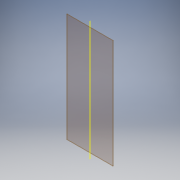
# Autodesk Inventor part: backOfRobot
Saved by Autodesk Inventor 2018.2 (Build 222227000, 227)
## iProperties
Created: 2018-02-09
Part Number: backOfRobot
Material: Polycarbonate, Smoke
Document SubType Name: Modeling
Designer: steele
Density: 1.2 g/cm^3
Appearance: Polycarbonate - Smoked
Author: steele
Autodesk Inventor part; units mm, degrees
ref_plane "XZ Plane" through (0, 0, 0) normal (0, 1, 0) x (-1, 0, 0)
ref_plane "XY Plane" through (0, 0, 0) normal (0, 0, 1) x (1, 0, 0)
sketch "Sketch1" plane through (0, 0, 0) normal (0, 0, 1) x (1, 0, 0)
  line L0 (-298.45, -698.5) -> (298.45, -698.5)
  line L1 (298.45, -698.5) -> (298.45, 698.5)
  line L2 (298.45, 698.5) -> (-298.45, 698.5)
  line L3 (-298.45, 698.5) -> (-298.45, -698.5)
  line L4 (-298.45, -698.5) -> (298.45, 698.5) construction
  line L5 (298.45, -698.5) -> (-298.45, 698.5) construction
  point P0 (0, 0)
  dimension "d0" = 596.9
  dimension "d1" = 1397
  constraints: 12 end point, 2 midpoint, 2 parallel, 1 horizontal, 1 perpendicular
  measures "d0" distance of L0.start L0.end
  measures "d1" distance of L1.end L0.end
extrude "Extrusion1" add sketch "Sketch1" along normal blind 6.35
body "Solid1"
